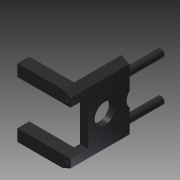
# Autodesk Inventor part: Back Support
Saved by Autodesk Inventor 2015 (Build 190159000, 159)
## iProperties
Created: 2015-11-29
Part Number: Back Support
Material: ABS Plastic
Document SubType Name: Modeling
Designer: James
Density: 1.06 g/cm^3
Appearance: Smooth - White
Mass: 22.3114 g
Surface Area: 106.088 cm^2
Volume: 21.0485 cm^3
Author: James
Autodesk Inventor part; units mm, degrees
ref_plane "YZ Plane" through (0, 0, 0) normal (1, 0, 0) x (0, 1, 0)
ref_plane "XZ Plane" through (0, 0, 0) normal (0, 1, 0) x (-1, 0, 0)
ref_plane "XY Plane" through (0, 0, 0) normal (0, 0, 1) x (1, 0, 0)
sketch "Sketch1" plane through (0, 0, 0) normal (0, 1, 0) x (-1, 0, 0)
  line L0 (0, 5) -> (0, 12)
  line L1 (0, 5) -> (7, 5)
  line L2 (7, 5) -> (7, 15)
  line L3 (7, 15) -> (0, 12)
  line L4 (0, -32.61) -> (7, -32.61)
  line L5 (7, -32.61) -> (7, -42.61)
  line L6 (0, -32.61) -> (0, -39.61)
  line L7 (0, -39.61) -> (7, -42.61)
  point P0 (0, 0)
  dimension "d2" = 5
  dimension "d3" = 7
  dimension "d5" = 7
  dimension "d6" = 10
  dimension "d7" = 7
  dimension "d8" = 10
  dimension "d9" = 7
  constraints: 16 end point, 2 point on line, 1 horizontal, 1 perpendicular, 1 vertical
  measures "d2" distance of point (0, 0) L0.start
  measures "d3" distance of L0.start L0.end
  measures "d5" distance of L0.start L1.end
  measures "d6" distance of L1.end L2.end
  measures "d7" distance of L4.start L4.end
  measures "d8" distance of L4.end L5.end
  measures "d9" distance of L4.start L6.end
extrude "Extrusion1" add sketch "Sketch1" along normal blind 15
sketch "Sketch2" plane through (0, 15, 0) normal (0, 1, 0) x (1, 0, 0)
  line L0 (-7, -15) -> (-7, 42.61)
  line L1 (-7, 42.61) -> (0, 39.61)
  line L2 (0, 39.61) -> (-7, 42.61) projected
  line L3 (0, 39.61) -> (0, -12)
  line L4 (0, -12) -> (-7, -15)
  point P0 (0, 0)
  constraints: 8 end point, 1 collinear, 1 parallel, 1 vertical
extrude "Extrusion2" add sketch "Sketch2" along normal blind 35
sketch "Sketch3" plane through (0, 50, 0) normal (0, 1, 0) x (1, 0, 0)
  line L0 (0, -12) -> (-7, -15) projected
  line L1 (-7, 42.61) -> (0, 39.61) projected
  circle A0 centre (-3.5, 31.11) radius 1.4
  circle A1 centre (-3.5, -3.5) radius 1.4
  circle A2 centre (-3.5, -3.5) radius 3.1
  circle A3 centre (-3.5, 31.11) radius 3.1
  point P0 (0, 0)
  dimension "d73" = 6.2
  dimension "d74" = 6.2
  constraints: 4 centre point, 2 coincident
  measures "d73" diameter of A2
  measures "d74" diameter of A3
sketch "Sketch4" plane through (0, 0, 0) normal (0, -1, 0) x (1, 0, 0)
  line L0 (0, 5) -> (0, 12) projected
  line L1 (0, 12) -> (-7, 15) projected
  line L2 (-7, 15) -> (-7, 5) projected
  line L3 (-7, 5) -> (0, 5) projected
  line L4 (0, -32.61) -> (-7, -32.61) projected
  line L5 (-7, -32.61) -> (-7, -42.61) projected
  line L6 (-7, -42.61) -> (0, -39.61) projected
  line L7 (0, -39.61) -> (0, -32.61) projected
  line L8 (-7, -42.61) -> (0, -32.61)
  line L9 (0, -39.61) -> (-7, -32.61)
  line L10 (0, 5) -> (-7, 15)
  line L11 (-7, 15) -> (0, 12)
  line L12 (0, 12) -> (-7, 5)
  circle A0 centre (-2.8824, 9.1176) radius 1.4
  circle A1 centre (-2.8824, -36.7276) radius 1.4
  point P0 (0, 0)
  dimension "d14" = 2.8
  dimension "d15" = 2.8
  constraints: 10 end point, 4 point on line, 2 centre point, 1 collinear, 1 perpendicular
  measures "d14" diameter of A0
  measures "d15" diameter of A1
extrude "Extrusion3" cut sketch "Sketch4" against normal blind 15 contours A0 L12 L10 | L10 L12 A0 | L12 L10 A0 | A0 L10 L12 | A1 L9 L8 | L8 L9 A1 | L9 L8 A1 | A1 L8 L9
extrude "Extrusion4" add sketch "Sketch3" along normal blind 30
sketch "Sketch6" plane through (-7, 0, -42.61) normal (-1, 0, 0) x (0, 0, 1)
  line L0 (10, 15) -> (47.61, 15) projected
  line L1 (28.805, 15) -> (28.805, 20)
  line L2 (28.805, 20) -> (38.805, 20)
  line L3 (38.805, 20) -> (38.805, 65)
  line L4 (38.805, 65) -> (18.805, 65)
  line L5 (18.805, 65) -> (18.805, 20)
  line L6 (18.805, 20) -> (28.805, 20)
  line L7 (18.805, 20) -> (18.805, 21.5)
  line L8 (18.805, 21.5) -> (20.305, 21.5)
  line L9 (38.805, 20) -> (38.805, 21.5)
  line L10 (38.805, 21.5) -> (37.305, 21.5)
  circle A0 centre (20.305, 21.5) radius 0.6
  circle A1 centre (37.305, 21.5) radius 0.6
  line L11 (28.805, 20) -> (28.805, 29)
  line L12 (28.805, 29) -> (28.805, 56)
  circle A2 centre (28.805, 29) radius 8.5
  circle A3 centre (28.805, 56) radius 8.5
  point P0 (42.61, 0)
  dimension "d26" = 5
  dimension "d27" = 10
  dimension "d28" = 45
  dimension "d29" = 20
  dimension "d30" = 1.5
  dimension "d31" = 1.5
  dimension "d32" = 1.5
  dimension "d33" = 1.5
  dimension "d34" = 1.2
  dimension "d35" = 1.2
  dimension "d36" = 9
  dimension "d37" = 27
  dimension "d38" = 17
  dimension "d39" = 17
  constraints: 24 end point, 5 perpendicular, 4 centre point, 4 coincident, 3 point on line, 3 vertical, 1 horizontal, 1 midpoint
  measures "d26" distance of L1.start L1.end
  measures "d27" distance of L1.end L2.end
  measures "d28" distance of L2.end L3.end
  measures "d29" distance of L3.end L4.end
  measures "d30" distance of L5.end L7.end
  measures "d31" distance of L7.end L8.end
  measures "d32" distance of L2.end L9.end
  measures "d33" distance of L9.end L10.end
  measures "d34" diameter of A0
  measures "d35" diameter of A1
  measures "d36" distance of L1.end L11.end
  measures "d37" distance of L11.end L12.end
  measures "d38" diameter of A2
  measures "d39" diameter of A3
extrude "Extrusion5" cut sketch "Sketch6" against normal through all contours A3 | A2 L12 L11 | L11 L12 A2
sketch "Sketch7" plane through (-7, 0, -42.61) normal (-1, 0, 0) x (0, 0, 1)
  line L0 (10, 15) -> (47.61, 15)
  line L1 (28.805, 15) -> (28.805, 20)
  line L2 (28.805, 20) -> (38.805, 20)
  line L3 (38.805, 20) -> (38.805, 65)
  line L4 (38.805, 65) -> (18.805, 65)
  line L5 (18.805, 65) -> (18.805, 20)
  line L6 (18.805, 20) -> (28.805, 20)
  line L7 (18.805, 20) -> (18.805, 21.5)
  line L8 (18.805, 21.5) -> (20.305, 21.5)
  line L9 (38.805, 20) -> (38.805, 21.5)
  line L10 (38.805, 21.5) -> (37.305, 21.5)
  circle A0 centre (20.305, 21.5) radius 0.9
  circle A1 centre (37.305, 21.5) radius 0.9
  line L11 (28.805, 20) -> (28.805, 29)
  line L12 (28.805, 29) -> (28.805, 56)
  circle A2 centre (28.805, 29) radius 8.5
  circle A3 centre (28.805, 56) radius 8.5
  point P0 (42.61, 0)
  point P1 (42.61, 0)
  dimension "d42" = 5
  dimension "d43" = 10
  dimension "d44" = 45
  dimension "d45" = 20
  dimension "d46" = 1.5
  dimension "d47" = 1.5
  dimension "d48" = 1.5
  dimension "d49" = 1.5
  dimension "d50" = 1.8
  dimension "d51" = 1.8
  dimension "d52" = 9
  dimension "d53" = 27
  dimension "d54" = 17
  dimension "d55" = 17
  constraints: 26 end point, 5 perpendicular, 4 centre point, 4 coincident, 3 point on line, 3 vertical, 1 horizontal, 1 midpoint
  measures "d42" distance of L1.start L1.end
  measures "d43" distance of L1.end L9.start
  measures "d44" distance of L9.start L3.end
  measures "d45" distance of L3.end L5.start
  measures "d46" distance of L6.start L8.start
  measures "d47" distance of L8.start L8.end
  measures "d48" distance of L9.start L9.end
  measures "d49" distance of L9.end L10.end
  measures "d50" diameter of A0
  measures "d51" diameter of A1
  measures "d52" distance of L1.end L11.end
  measures "d53" distance of L11.end L12.end
  measures "d54" diameter of A2
  measures "d55" diameter of A3
extrude "Extrusion6" cut sketch "Sketch7" against normal blind 5 contours A1 | A0
sketch "Sketch8" plane through (-7, 0, -42.61) normal (-1, 0, 0) x (0, 0, 1)
  circle A0 centre (20.305, 21.5) radius 0.9 projected
  line L0 (20.305, 21.5) -> (20.305, 20)
  line L1 (20.305, 20) -> (18.805, 20)
  line L2 (18.805, 20) -> (18.805, 19)
  line L3 (18.805, 19) -> (17.805, 19)
  line L4 (17.805, 19) -> (39.805, 19)
  line L5 (39.805, 19) -> (39.805, 66)
  line L6 (39.805, 66) -> (17.805, 66)
  line L7 (17.805, 66) -> (17.805, 19)
  point P0 (42.61, 0)
  dimension "d58" = 1.5
  dimension "d59" = 1.5
  dimension "d60" = 1
  dimension "d61" = 1
  dimension "d62" = 22
  dimension "d63" = 47
  constraints: 16 end point, 4 perpendicular, 2 parallel, 1 point on line, 1 vertical
  measures "d58" distance of L0.start L0.end
  measures "d59" distance of L0.end L1.end
  measures "d60" distance of L1.end L2.end
  measures "d61" distance of L2.end L3.end
  measures "d62" distance of L3.end L4.end
  measures "d63" distance of L5.end L4.end
extrude "Extrusion7" cut sketch "Sketch8" against normal blind 2
sketch "Sketch9" plane through (-7, 0, -42.61) normal (-1, 0, 0) x (0, 0, 1)
  line L0 (10, 0) -> (0, 0)
  line L1 (0, 0) -> (0, 10)
  line L2 (0, 10) -> (10, 10)
  line L3 (10, 10) -> (10, 0)
  line L4 (47.61, 0) -> (57.61, 0)
  line L5 (57.61, 0) -> (57.61, 10)
  line L6 (57.61, 10) -> (47.61, 10)
  line L7 (47.61, 10) -> (47.61, 0)
  line L8 (57.61, 0) -> (47.61, 0) projected
  point P0 (42.61, 0)
  dimension "d66" = 10
  dimension "d67" = 10
  constraints: 16 end point, 5 equal length, 2 perpendicular, 1 horizontal
  measures "d66" distance of L0.end L1.end
  measures "d67" distance of L5.end L4.end
extrude "Extrusion8" add sketch "Sketch9" along normal blind 40
chamfer "Chamfer1" distance 2 angle 45 8 edges at (-47, 5, -42.61) (-47, 0, -37.61) (-47, 5, -32.61) (-47, 10, -37.61) (-47, 0, 10) (-47, 5, 15) (-47, 5, 5) (-47, 10, 10)
body "Solid1"
